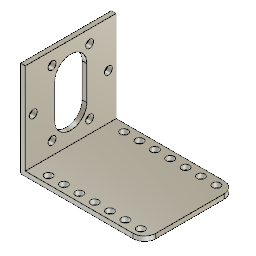
Motor holder (Autodesk Fusion 360 design; units mm, degrees)
Autodesk Fusion 360 part; units mm, degrees
sketch "Esquisse1" plane through (0, 0, 0) normal (0, 0, 1) x (1, 0, 0)
  line L0 (0, 0) -> (44.5, 0)
  line L1 (49.2, 4.7) -> (49.2, 32.9)
  line L2 (44.5, 37.6) -> (0, 37.6)
  line L3 (0, 37.6) -> (0, 0)
  line L4 (0, 37.6) -> (-2, 37.6)
  line L5 (-2, 37.6) -> (-2, 0)
  line L6 (-2, 0) -> (0, 0)
  line L7 (0, 0) -> (0, 37.6)
  circle A0 centre (6.4, 34.4) radius 1.6
  circle A1 centre (6.4, 3.2) radius 1.6
  circle A2 centre (38.1, 34.4) radius 1.6
  circle A3 centre (44.5, 34.4) radius 1.6
  circle A4 centre (38.1, 3.2) radius 1.6
  circle A5 centre (44.5, 3.2) radius 1.6
  arc A6 (49.2, 32.9) -> (44.5, 37.6) centre (44.5, 32.9) ccw
  arc A7 (44.5, 0) -> (49.2, 4.7) centre (44.5, 4.7) ccw
  circle A8 centre (12.74, 3.2) radius 1.6
  circle A9 centre (19.08, 3.2) radius 1.6
  circle A10 centre (25.42, 3.2) radius 1.6
  circle A11 centre (31.76, 3.2) radius 1.6
  circle A12 centre (12.74, 34.4) radius 1.6
  circle A13 centre (19.08, 34.4) radius 1.6
  circle A14 centre (25.42, 34.4) radius 1.6
  circle A15 centre (31.76, 34.4) radius 1.6
  point P0 (49.2, 0)
  dimension "d1" = 49.2
  dimension "d2" = 37.6
  dimension "d3" = 2
  dimension "d6" = 3.2
  dimension "d7" = 8.4
  dimension "d8" = 3.2
  dimension "d10" = 3.2
  dimension "d11" = 3.2
  dimension "d12" = 8.4
  dimension "d19" = 3.2
  dimension "d20" = 3.2
  dimension "d25" = 3.2
  dimension "d26" = 3.2
  dimension "d27" = 4.7
  dimension "d28" = 4.7
  dimension "d29" = 6.4
  dimension "d30" = 6.4
  dimension "d31" = 4.7
  dimension "d32" = 4.7
  dimension "d48" = 3.2
  dimension "d49" = 3.2
  dimension "d50" = 3.2
  dimension "d51" = 3.2
  dimension "d52" = 3.2
  dimension "d53" = 3.2
  dimension "d54" = 3.2
  dimension "d55" = 3.2
  constraint horizontal L0
  constraint vertical L1
  constraint horizontal L2
  constraint vertical L3
  constraint coincident L0.start L3.end
  constraint horizontal L4
  constraint vertical L5
  constraint horizontal L6
  constraint vertical L7
  constraint tangent L2 A6
  constraint tangent L1 A6
  constraint coincident P0 L0
  constraint coincident P0 L1
  constraint tangent L0 A7
  constraint tangent L1 A7
  measures "d1" distance of L0.start P0
  measures "d2" distance of L0.start L2.end
  measures "d3" distance of L2.end L4.end
  measures "d6" diameter of A0
  measures "d7" distance of L5 A0.centre
  measures "d8" diameter of A1
  measures "d10" distance of L2 A0.centre
  measures "d11" distance of L0 A1.centre
  measures "d12" distance of L5 A1.centre
  measures "d19" diameter of A2
  measures "d20" diameter of A3
  measures "d25" diameter of A4
  measures "d26" diameter of A5
  measures "d27" distance of L1 A3.centre
  measures "d28" distance of L1 A5.centre
  measures "d29" distance of A2.centre A3.centre
  measures "d30" distance of A5.centre A4.centre
  measures "d31" radius of A6
  measures "d32" radius of A7
  measures "d48" diameter of A8
  measures "d49" diameter of A9
  measures "d50" diameter of A10
  measures "d51" diameter of A11
  measures "d52" diameter of A12
  measures "d53" diameter of A13
  measures "d54" diameter of A14
  measures "d55" diameter of A15
extrude "Extrusion1" add sketch "Esquisse1" along normal blind 2 contours L0 L1 L2 L3 L7 A6 A7 | L3 L4 L5 L6 L7 | A0 | A1 | A2 | A3 | A4 | A5 | A8 | A9 | A10 | A11 | A12 | A13 | A14 | A15 makes body 1
extrude "Extrusion3" add sketch "Esquisse1" along normal blind 39.6 contours L3 L4 L5 L6 L7 bodies 1
sketch "Esquisse2" plane through (-2, 0, 0) normal (-1, 0, 0) x (0, -1, 0)
  line L0 (-37.6, 0) -> (0, 0)
  line L1 (0, 0) -> (0, 39.6)
  line L2 (0, 39.6) -> (-37.6, 39.6)
  line L3 (-37.6, 39.6) -> (-37.6, 0)
  circle A0 centre (-3.3, 20.8) radius 1.65
  circle A1 centre (-11.05, 34.2234) radius 1.65
  circle A2 centre (-26.55, 34.2234) radius 1.65
  circle A3 centre (-34.3, 20.8) radius 1.65
  circle A4 centre (-26.55, 7.3766) radius 1.65
  circle A5 centre (-11.05, 7.3766) radius 1.65
  line L4 (-25.4, 27.8) -> (-25.4, 13.8)
  line L5 (-12.2, 13.8) -> (-12.2, 27.8)
  line L6 (-12.2, 27.8) -> (-25.4, 13.8) construction
  line L7 (-25.4, 27.8) -> (-12.2, 13.8) construction
  arc A6 (-12.2, 27.8) -> (-25.4, 27.8) centre (-18.8, 27.8) ccw
  arc A7 (-25.4, 13.8) -> (-12.2, 13.8) centre (-18.8, 13.8) ccw
  arc A8 (-18.8, 39.6) -> (-37.6, 20.8) centre (-18.8, 20.8) ccw
  arc A9 (0, 20.8) -> (-18.8, 39.6) centre (-18.8, 20.8) ccw
  point P0 (-18.8, 20.8)
  dimension "d39" = 3.3
  dimension "d42" = 13.2
  dimension "d43" = 14
  constraint parallel L4 L5
  constraint coincident L6 P0
  constraint coincident L7 P0
  constraint coincident L2 A8.start
  constraint coincident L3 A8.end
  constraint coincident P0 A8.centre
  constraint coincident L1 A9.start
  measures "d39" diameter of A0
  measures "d42" distance of L4.end L5.start
  measures "d43" distance of L4.start L4.end
extrude "Extrusion4" cut sketch "Esquisse2" against normal blind 19 contours A0 | A1 | A2 | A3 | A4 | A5 | L4 L5 A6 A7 bodies 1
extrude "Extrusion5" cut sketch "Esquisse1" along normal blind 8 contours A0 | A1 | A2 | A3 | A4 | A5 | A8 | A9 | A10 | A11 | A12 | A13 | A14 | A15 bodies 1
copy_body "Corps->Comp3" bodies 1 removing the originals makes body 2 in component "Component"
component "Component" placed x (1, 0, 0) y (0, 1, 0) z (0, 0, 1) at (0, 0, 0)
